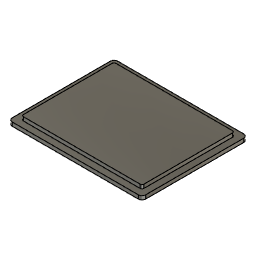
DisplayCaseGlas (Autodesk Fusion 360 design; units mm, degrees)
Autodesk Fusion 360 part; units mm, degrees
sketch "Skizze1" plane through (0, 0, 0) normal (0, 0, 1) x (1, 0, 0)
  line L0 (0, 0) -> (18.1, 0)
  line L1 (18.1, 0) -> (18.1, 14.3)
  line L2 (18.1, 14.3) -> (0, 14.3)
  line L3 (0, 14.3) -> (0, 0)
  dimension "d1" = 18.1
  dimension "d2" = 14.3
  constraint horizontal L0
  constraint vertical L1
  constraint horizontal L2
  constraint vertical L3
  constraint coincident L0.start L3.end
  measures "d1" distance of L0.start L0.end
  measures "d2" distance of L0.end L1.end
extrude "Extrusion1" add sketch "Skizze1" along normal blind 2
sketch "Skizze2" plane through (0, 0, 2) normal (0, 0, 1) x (-1, 0, 0)
  line L0 (0, 0) -> (-16.35, 0)
  line L1 (-16.35, 0) -> (-16.35, -12.55)
  line L2 (-16.35, -12.55) -> (0, -12.55)
  line L3 (0, -12.55) -> (0, 0)
  line L4 (0, -14.3) -> (0, 0)
  line L5 (0, 0) -> (-18.1, 0)
  line L6 (-18.1, 0) -> (-18.1, -14.3)
  line L7 (-18.1, -14.3) -> (0, -14.3)
  point P0 (-18.1, 0)
  point P1 (0, -14.3)
  dimension "d19" = 16.35
  dimension "d20" = 12.55
  constraint horizontal L0
  constraint vertical L1
  constraint horizontal L2
  constraint vertical L3
  constraint coincident L0.start L3.end
  measures "d19" distance of L0.start L0.end
  measures "d20" distance of L0.end L1.end
extrude "Extrusion2" cut sketch "Skizze2" against normal blind 1 contours L1 L2 L4 L5 L6 L7
mirror "Spiegeln1" about plane through (0, 14.3, 0) normal (-1, 0, 0) of bodies 1 merged
mirror "Spiegeln2" about plane through (0, 0, 0) normal (0, 1, 0) of bodies 1 merged
fillet "Abrundung1" radius 0.5 4 edges at (-16.35, -12.55, 1.5) (-16.35, 12.55, 1.5) (16.35, 12.55, 1.5) (16.35, -12.55, 1.5)
fillet "Abrundung1" radius 1 4 edges at (-18.1, -14.3, 0.5) (-18.1, 14.3, 0.5) (18.1, 14.3, 0.5) (18.1, -14.3, 0.5)
equation "d1 = ( ( 37.6 - 0.5 ) / 2 ) * 1 mm - 0.45 mm"
equation "d2 = ( ( 30 - 0.5 ) / 2 ) * 1 mm - 0.45 mm"
equation "d19 = ( ( 33.6 - 0.5 ) / 2 ) * 1 mm - 0.2 mm"
equation "d20 = ( ( 26 - 0.5 ) / 2 ) * 1 mm - 0.2 mm"
